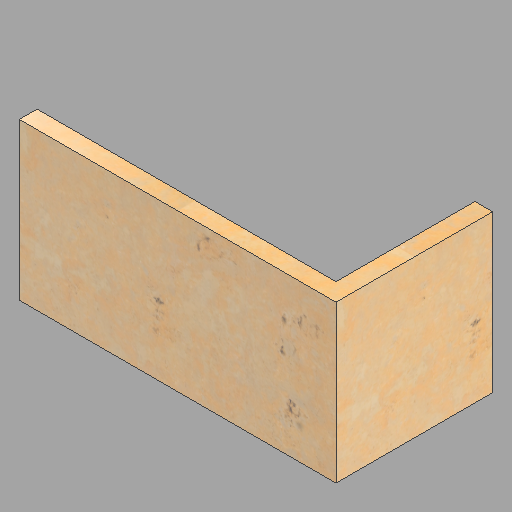
# Autodesk Inventor part: Corner
Saved by Autodesk Inventor 2023 (Build 270158030, 158C)
## iProperties
RuleStatus: InUse
Created: 2022-03-23
Part Number: Corner
Material: Granite, Cut, Polished
Document SubType Name: Modeling
Designer: awelt
Mass: 79931.5 g
Surface Area: 13432.6 cm^2
Volume: 29604.3 cm^3
Density: 2.7 g/cm^3
Appearance: Amber Select
AfterDocSave0: Convert in3 volume to ft3
in3 to ft3: 1.05
TEST: 1.045
Author: awelt
Autodesk Inventor part; units mm, degrees
ref_plane "YZ Plane" through (0, 0, 0) normal (1, 0, 0) x (0, 1, 0)
ref_plane "XZ Plane" through (0, 0, 0) normal (0, 1, 0) x (-1, 0, 0)
ref_plane "XY Plane" through (0, 0, 0) normal (0, 0, 1) x (1, 0, 0)
sketch "Sketch1" plane through (0, 0, 0) normal (0, 1, 0) x (-1, 0, 0)
  line L0 (0, 0) -> (904.875, 0)
  line L1 (904.875, 0) -> (904.875, -50.8)
  line L2 (0, 0) -> (0, -447.675)
  line L3 (0, -447.675) -> (50.8, -447.675)
  line L4 (50.8, -447.675) -> (50.8, -50.8)
  line L5 (50.8, -50.8) -> (904.875, -50.8)
  dimension "d0" = 904.875
  dimension "d1" = 50.8
  dimension "d2" = 447.675
  dimension "d3" = 50.8
  constraints: 12 end point, 3 perpendicular, 1 horizontal, 1 parallel, 1 vertical
  measures "d0" distance of L0.start L0.end
  measures "d1" distance of L0.end L1.end
  measures "d2" distance of L0.start L2.end
  measures "d3" distance of L2.end L3.end
extrude "Extrusion1" add sketch "Sketch1" along normal blind 447.675
body "Solid1"
